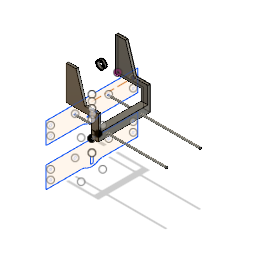
chariot (Autodesk Fusion 360 design; units mm, degrees)
Autodesk Fusion 360 part; units mm, degrees
note: some values were not read from the file. Set by a fixed rule: which face or edge a step refers to.
sketch "Sketch1" plane through (0, 0, 0) normal (0, 0, 1) x (1, 0, 0)
  line L0 (0, 111.6) -> (0, 0)
  line L1 (0, 111.6) -> (32.8, 111.6)
  line L2 (0, 0) -> (83.35, 0)
  line L3 (83.35, 0) -> (83.35, -60.4)
  line L4 (83.35, -60.4) -> (106.05, -60.4)
  line L5 (106.05, -60.4) -> (106.05, 19.85)
  line L6 (106.05, 19.85) -> (61.2, 19.85)
  line L7 (32.8, 111.6) -> (61.2, 19.85)
  dimension "d1" = 111.6
  dimension "d2" = 32.8
  dimension "d3" = 83.35
  dimension "d5" = 22.7
  dimension "d6" = 80.25
  dimension "d7" = 44.85
  dimension "d10" = 19.85
  constraint coincident L0.end L2.start
  constraint vertical L0
  constraint perpendicular L0 L1
  constraint perpendicular L0 L2
  constraint perpendicular L2 L3
  constraint perpendicular L3 L4
  constraint perpendicular L4 L5
  constraint perpendicular L5 L6
  measures "d1" distance of L0.start L0.end
  measures "d2" distance of L0.start L1.end
  measures "d3" distance of L0.end L2.end
  measures "d5" distance of L3.end L4.end
  measures "d6" distance of L4.end L5.end
  measures "d7" distance of L5.end L6.end
  measures "d10" distance of L2 L6
extrude "Extrude1" add sketch "Sketch1" along normal blind 8 makes body 1
copy_body "CopyPasteBodies1" bodies 1 makes body 2
move_body "Move1" bodies 2 to x (1, 0, 0) y (0, 1, 0) z (0, 0, 1) at (0, 0, 162)
sketch "Sketch2" plane through (0, 0, 170) normal (0, 0, 1) x (1, 0, 0)
  line L0 (0, 111.6) -> (0, 0)
  line L1 (0, 0) -> (83.35, 0)
  line L2 (83.35, 0) -> (83.35, -60.4)
  line L3 (83.35, -60.4) -> (106.05, -60.4)
  line L4 (106.05, -60.4) -> (106.05, 19.85)
  line L5 (106.05, 19.85) -> (61.2, 19.85)
  line L6 (61.2, 19.85) -> (32.8, 111.6)
  line L7 (32.8, 111.6) -> (0, 111.6)
  line L8 (83.35, -60.4) -> (83.35, -35.4)
  line L9 (83.35, -35.4) -> (106.05, -35.4)
  dimension "d11" = 25
  constraint coincident L2.end L3.start
  constraint perpendicular L3 L8
  constraint coincident L4 L9.end
  constraint perpendicular L4 L9
  measures "d11" distance of L2.end L8.end
extrude "Extrude2" add sketch "Sketch2" against normal blind 162 contours L2 L3 L4 L8 L9 bodies 2 1
cylinder "CylinderPrimitive1" add diameter 8 height 300 placed x (0, 0, -1) y (0, 1, 0) z (1, 0, 0) at (0, 0, 100) separate body makes body 3
move_body "Move2" bodies 3 to x (1, 0, 0) y (0, 1, 0) z (0, 0, 1) at (0, -50, 40)
copy_body "CopyPasteBodies2" bodies 3 makes body 4
move_body "Move3" bodies 4 to x (1, 0, 0) y (0, 1, 0) z (0, 0, 1) at (0, 0, -110)
sketch "Sketch4" plane through (0, 0, 0) normal (1, 0, 0) x (0, 0, -1)
  line L0 (65, -20) -> (-85, -20)
  line L1 (-49.6312, -90) -> (65, -90)
  line L2 (65, -90) -> (65, -40)
  line L3 (-235, -20) -> (-85, -20)
  line L4 (-235, -90) -> (-235, -20)
  line L5 (-120.4495, -90) -> (-235, -90)
  line L6 (-85, -40) -> (65, -40) construction
  circle A0 centre (50, -40) radius 3.25
  circle A1 centre (50, -70) radius 3.25
  circle A2 centre (-220, -40) radius 4
  circle A3 centre (-220, -70) radius 4
  circle A4 centre (-29.9081, -47.5) radius 3.9717
  circle A5 centre (-140.0919, -47.5) radius 3.9717
  line L7 (65, -40) -> (65, -20)
  line L8 (-85, -61.1344) -> (-80.5, -61.1344)
  line L9 (-80.5, -91.1344) -> (-85, -91.1344)
  line L10 (-85, -61.1344) -> (-89.5, -61.1344)
  line L11 (-89.5, -91.1344) -> (-85, -91.1344)
  line L12 (-70, -74.0844) -> (-80.5, -74.0844)
  line L13 (-80.5, -78.1844) -> (-70, -78.1844)
  line L14 (-70, -78.1844) -> (-70, -74.0844)
  arc A6 (-103.718, -94.2583) -> (-66.3628, -94.2583) centre (-85.0404, -59.941) ccw
  arc A7 (-49.6312, -90) -> (-66.3628, -94.2583) centre (-49.6312, -125) ccw
  arc A8 (-103.718, -94.2583) -> (-120.4495, -90) centre (-120.4495, -125) ccw
  line L15 (-235, -145) -> (-85, -145)
  line L16 (-235, -215) -> (-235, -145)
  line L17 (-120.4495, -215) -> (-235, -215)
  arc A9 (-103.718, -219.2583) -> (-120.4495, -215) centre (-120.4495, -250) ccw
  arc A10 (-103.718, -219.2583) -> (-66.3628, -219.2583) centre (-85.0404, -184.941) ccw
  arc A11 (-49.6312, -215) -> (-66.3628, -219.2583) centre (-49.6312, -250) ccw
  line L18 (-49.6312, -215) -> (65, -215)
  line L19 (65, -215) -> (65, -165)
  line L20 (65, -165) -> (65, -145)
  line L21 (65, -145) -> (-85, -145)
  circle A12 centre (50, -165) radius 3.25
  circle A13 centre (50, -195) radius 3.25
  circle A14 centre (-29.9081, -172.5) radius 3.9717
  circle A15 centre (-140.0919, -172.5) radius 3.9717
  circle A16 centre (-220, -165) radius 3.25
  circle A17 centre (-220, -195) radius 3.25
  line L22 (-85, -186.1344) -> (-80.5, -186.1344)
  line L23 (-80.5, -216.1344) -> (-85, -216.1344)
  line L24 (-80.5, -186.1344) -> (-80.5, -216.1344)
  line L25 (-85, -186.1344) -> (-89.5, -186.1344)
  line L26 (-89.5, -216.1344) -> (-85, -216.1344)
  line L27 (-89.5, -186.1344) -> (-89.5, -216.1344)
  line L28 (-82.75, -74.0844) -> (-82.75, -78.1844) construction
  line L29 (-89.5, -78.1844) -> (-100, -78.1844)
  line L30 (-100, -78.1844) -> (-100, -74.0844)
  line L31 (-100, -74.0844) -> (-89.5, -74.0844)
  line L32 (-89.5, -61.1344) -> (-89.5, -74.0844)
  line L33 (-89.5, -78.1844) -> (-89.5, -91.1344)
  line L34 (-80.5, -61.1344) -> (-80.5, -74.0844)
  line L35 (-80.5, -78.1844) -> (-80.5, -91.1344)
  dimension "d17" = 6.5
  dimension "d19" = 4.5
  dimension "d20" = 30
  dimension "d22" = 4.1
  dimension "d23" = 35
  dimension "d37" = 6.5
  dimension "d38" = 4.5
  dimension "d39" = 30
  dimension "d40" = 35
  dimension "d41" = 6.5
  dimension "d42" = 6.5
  dimension "d43" = 6.5
  constraint horizontal L0
  constraint perpendicular L0 L2
  constraint perpendicular L1 L2
  constraint coincident L6 A0.centre
  constraint perpendicular L0 L7
  constraint perpendicular L8 L34
  constraint horizontal L12
  constraint horizontal L13
  constraint vertical L14
  constraint tangent A6 A7
  constraint tangent L1 A7
  constraint tangent A6 A8
  constraint tangent L5 A8
  constraint equal A7 A8
  constraint horizontal L21
  constraint perpendicular L19 L21
  constraint perpendicular L18 L19
  constraint perpendicular L20 L21
  constraint perpendicular L22 L24
  constraint tangent A10 A11
  constraint tangent A11 L18
  constraint tangent A9 A10
  constraint tangent L17 A9
  constraint equal A9 A11
  constraint coincident L13.start L34
  constraint coincident L23.end L26.end
  measures "d17" diameter of A0
  measures "d19" distance of L8.start L8.end
  measures "d20" distance of L8.end L9.start
  measures "d22" distance of L12.start L13.end
  measures "d23" radius of A7
  measures "d37" diameter of A12
  measures "d38" distance of L22.end L22.start
  measures "d39" distance of L22.end L23.start
  measures "d40" radius of A11
  measures "d41" diameter of A13
  measures "d42" diameter of A16
  measures "d43" diameter of A17
sketch "Sketch5" plane through (0, 0, 0) normal (0, 0, 1) x (1, 0, 0)
  circle A0 centre (-50, 0) radius 11.05
  circle A1 centre (-50, 0) radius 12.75
  circle A2 centre (-50, 0) radius 14
  circle A3 centre (-50, 0) radius 11.675
  dimension "d24" = 22.1
  dimension "d25" = 25.5
  dimension "d26" = 28
  dimension "d31" = 0.625
  dimension "d32" = 1.25
  constraint concentric A0 A1
  constraint concentric A0 A2
  constraint concentric A2 A3
  measures "d24" diameter of A0
  measures "d25" diameter of A1
  measures "d26" diameter of A2
  measures "d31" distance of A0 A3
extrude "Extrude3" add sketch "Sketch5" along normal blind 7.5 separate body contours A1 | A3 makes body 5
extrude "Extrude4" add sketch "Sketch5" along normal blind 0.75 contours A1 | A2 | A3 bodies 5
extrude "Extrude5" add sketch "Sketch5" along normal blind 0.75 separate body contours A1 | A2 makes body 6
move_body "Move4" bodies 6 to x (1, 0, 0) y (0, 1, 0) z (0, 0, 1) at (0, 0, 6.75)
copy_body "CopyPasteBodies3" bodies 6 makes body 7
combine "Combine1" operation cut target body 5 tool bodies 7
move_face "MoveFace1" by (0, 0, 0.2) 1 faces at (-59.765, 5.9557, 7.5) on bodies 5
chamfer "Chamfer1" distance 0.2 angle 45 1 edges at (-60.8849, -4.2219, 7.7) on bodies 5
move_face "MoveFace2" by (0, 0, 0.5) 1 faces at (-59.9251, -5.4124, 7.7) on bodies 5
move_body "Move5" bodies 6 to x (1, 0, 0) y (0, 1, 0) z (0, 0, 1) at (0, 0, 1)
move_face "OffsetFaces1" offset -0.15 1 faces at (-38.3395, 0.582, 7.1667) on bodies 5
move_body "Move6" bodies 6 to x (1, 0, 0) y (0, 1, 0) z (0, 0, 1) at (0, 0, -1)
move_face "MoveFace3" by (0, 0, 1) 1 faces at (-36.8271, -0.6955, 7.5) on bodies 6
move_face "MoveFace4" by (0, 0, 1) 1 faces at (-36.8271, 0.6955, 8.5) on bodies 6
move_face "MoveFace5" by (0, 0, -2) 1 faces at (-37.0766, 1.2445, 0) on bodies 5
move_face "MoveFace6" by (0, 0, 1.3) 1 faces at (-60.5281, -3.8363, 8.2) on bodies 5
equation "d3 = 105.25 mm - 21.90 mm"
equation "d6 = 60.25 mm + 20 mm"
equation "d19 = ( ( 7 / 2 ) * 1 mm ) + 1 mm"
equation "d25 = 23 mm + 2.5 mm"
equation "d31 = ( 1.25 / 2 ) * 1 mm"
equation "d38 = ( ( 7 / 2 ) * 1 mm ) + 1 mm"
equation "d39 = d20"
equation "d41 = d37"
equation "d42 = d37"
equation "d43 = d37"
